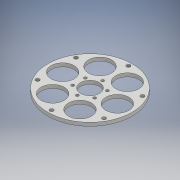
# Autodesk Inventor part: SprocketHubPlate
Saved by Autodesk Inventor 2019.3 (Build 233278000, 278)
## iProperties
Created: 2017-05-06
Part Number: SprocketHubPlate
Material: Generic
Document SubType Name: Modeling
Designer: eroldan
Density: 1 g/cm^3
Appearance: Default
Author: eroldan
Autodesk Inventor part; units mm, degrees
ref_plane "YZ Plane" through (0, 0, 0) normal (1, 0, 0) x (0, 1, 0)
ref_plane "XZ Plane" through (0, 0, 0) normal (0, 1, 0) x (-1, 0, 0)
ref_plane "XY Plane" through (0, 0, 0) normal (0, 0, 1) x (1, 0, 0)
sketch "Sketch1" plane through (0, 0, 0) normal (0, 0, 1) x (1, 0, 0)
  circle A0 centre (0, 0) radius 16.5
  circle A1 centre (-47.5262, 0) radius 20
  circle A2 centre (0, 0) radius 73
  circle A3 centre (-23.7631, -41.1589) radius 20
  circle A4 centre (23.7631, -41.1589) radius 20
  circle A5 centre (47.5262, 0) radius 20
  circle A6 centre (23.7631, 41.1589) radius 20
  circle A7 centre (-23.7631, 41.1589) radius 20
  point P0 (0, 66.675)
  point P1 (-57.7422, 33.3375)
  point P2 (-57.7422, -33.3375)
  point P3 (0, -66.675)
  point P4 (57.7422, -33.3375)
  point P5 (57.7422, 33.3375)
  point P6 (0, 22)
  point P7 (-19.0526, 11)
  point P8 (-19.0526, -11)
  point P9 (0, -22)
  point P10 (19.0526, -11)
  point P11 (19.0526, 11)
  dimension "d0" = 66.675
  dimension "d3" = 360
  dimension "d9" = 33
  dimension "d19" = 40
  dimension "d20" = 22
  dimension "d23" = 360
  dimension "d25" = 146
  dimension "d28" = 360
  constraints: 8 centre point, 1 coincident, 27 other
  measures "d0" distance of point (0, 0) point (0, 66.675)
  measures "d9" diameter of A0
  measures "d19" diameter of A1
  measures "d20" distance of point (0, 22) point (0, 0)
  measures "d25" diameter of A2
extrude "Extrusion2" add sketch "Sketch1" along normal blind 6
hole "Hole2" at (0, 66.675, 0) at (-57.7422, 33.3375, 0) at (-57.7422, -33.3375, 0) at (0, -66.675, 0) at (57.7422, -33.3375, 0) at (57.7422, 33.3375, 0) direction (0, 0, 1) diameter 6.5 end through all
hole "Hole3" at (0, 22, 0) at (-19.0526, 11, 0) at (-19.0526, -11, 0) at (0, -22, 0) at (19.0526, 11, 0) at (19.0526, -11, 0) direction (0, 0, 1) diameter 5 end through all
